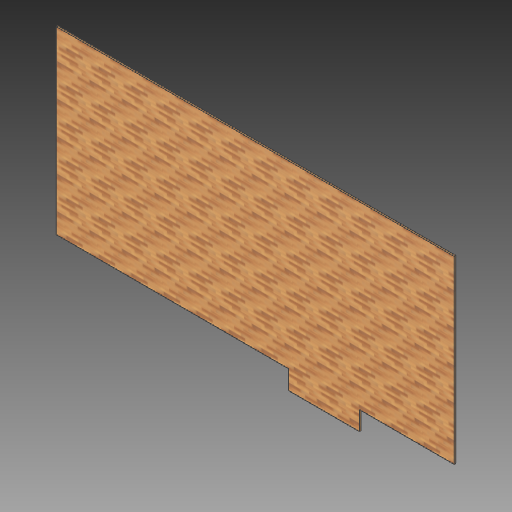
# Autodesk Inventor part: Пол гостиной
Saved by Autodesk Inventor 2019 (Build 230136000, 136)
## iProperties
Created: 2018-09-19
Part Number: Пол гостиной
Material: Деревянные полы
Document SubType Name: Modeling
Designer: Андреев Н.Л.
Density: 0.673 g/cm^3
Appearance: Бук — гальяно
Author: Андреев Н.Л.
Autodesk Inventor part; units mm, degrees
ref_plane "YZ Plane" through (0, 0, 0) normal (1, 0, 0) x (0, 1, 0)
ref_plane "XZ Plane" through (0, 0, 0) normal (0, 1, 0) x (-1, 0, 0)
ref_plane "XY Plane" through (0, 0, 0) normal (0, 0, 1) x (1, 0, 0)
sketch "Эскиз1" plane through (0, 0, 0) normal (0, 0, 1) x (1, 0, 0)
  line L0 (23007.3162, 20272.69) -> (23007.3162, 20672.69) construction
  line L1 (25007.3162, 20672.69) -> (23007.3162, 20672.69) construction
  line L2 (25007.3162, 20272.69) -> (25007.3162, 20672.69) construction
  line L3 (23007.3162, 20272.69) -> (25007.3162, 20272.69) construction
  line L4 (21507.3162, 20672.69) -> (21507.3162, 20272.69) construction
  line L5 (19507.3162, 20272.69) -> (21507.3162, 20272.69) construction
  line L6 (19507.3162, 20672.69) -> (19507.3162, 20272.69) construction
  line L7 (21507.3162, 20672.69) -> (19507.3162, 20672.69) construction
  line L8 (28307.3162, 15072.69) -> (28307.3162, 14672.69) construction
  line L9 (27607.3162, 14672.69) -> (28307.3162, 14672.69) construction
  line L10 (27607.3162, 15072.69) -> (27607.3162, 14672.69) construction
  line L11 (26657.3162, 15072.69) -> (27607.3162, 15072.69) construction
  line L12 (26657.3162, 15072.69) -> (26657.3162, 15472.69) construction
  line L13 (27607.3162, 15472.69) -> (26657.3162, 15472.69) construction
  line L14 (27607.3162, 23072.69) -> (27607.3162, 15472.69) construction
  line L15 (25407.3162, 23072.69) -> (27607.3162, 23072.69) construction
  line L16 (25407.3162, 20072.69) -> (25407.3162, 23072.69) construction
  line L17 (25407.3162, 20072.69) -> (25007.3162, 20072.69) construction
  line L18 (25007.3162, 14072.69) -> (25007.3162, 17872.69) construction
  line L19 (25007.3162, 24472.69) -> (16607.3162, 24472.69) construction
  line L20 (16607.3162, 24472.69) -> (16607.3162, 20672.69) construction
  line L21 (19507.3162, 20672.69) -> (16607.3162, 20672.69) construction
  line L22 (19507.3162, 20272.69) -> (19507.3162, 20672.69) construction
  line L23 (16607.3162, 20272.69) -> (19507.3162, 20272.69) construction
  line L24 (16607.3162, 20272.69) -> (16607.3162, 18272.69) construction
  line L25 (19607.3162, 18272.69) -> (16607.3162, 18272.69) construction
  line L26 (19607.3162, 18272.69) -> (19607.3162, 17872.69) construction
  line L27 (16607.3162, 17872.69) -> (19607.3162, 17872.69) construction
  line L28 (16607.3162, 17872.69) -> (16607.3162, 14072.69) construction
  line L29 (16607.3162, 14072.69) -> (25007.3162, 14072.69) construction
  line L30 (23857.3162, 17872.69) -> (25007.3162, 17872.69) construction
  line L31 (23857.3162, 17872.69) -> (23857.3162, 18272.69) construction
  line L32 (25007.3162, 18272.69) -> (23857.3162, 18272.69) construction
  line L33 (25007.3162, 18272.69) -> (25007.3162, 18572.69) construction
  line L34 (25007.3162, 18572.69) -> (25407.3162, 18572.69) construction
  line L35 (25407.3162, 15472.69) -> (25407.3162, 18572.69) construction
  line L36 (25657.3162, 15472.69) -> (25407.3162, 15472.69) construction
  line L37 (25657.3162, 15472.69) -> (25657.3162, 15072.69) construction
  line L38 (25407.3162, 15072.69) -> (25657.3162, 15072.69) construction
  line L39 (25407.3162, 13672.69) -> (25407.3162, 15072.69) construction
  line L40 (16207.3162, 13672.69) -> (25407.3162, 13672.69) construction
  line L41 (16207.3162, 15072.69) -> (16207.3162, 13672.69) construction
  line L42 (15957.3162, 15072.69) -> (16207.3162, 15072.69) construction
  line L43 (15957.3162, 15072.69) -> (15957.3162, 15472.69) construction
  line L44 (16207.3162, 15472.69) -> (15957.3162, 15472.69) construction
  line L45 (16207.3162, 23472.69) -> (16207.3162, 15472.69) construction
  line L46 (14007.3162, 23472.69) -> (16207.3162, 23472.69) construction
  line L47 (14007.3162, 20472.69) -> (14007.3162, 23472.69) construction
  line L48 (14007.3162, 20472.69) -> (13607.3162, 20472.69) construction
  line L49 (13607.3162, 20472.69) -> (13607.3162, 23472.69) construction
  line L50 (13607.3162, 23472.69) -> (8007.3162, 23472.69) construction
  line L51 (8007.3162, 23472.69) -> (8007.3162, 15072.69) construction
  line L52 (8007.3162, 15072.69) -> (13607.3162, 15072.69) construction
  line L53 (13607.3162, 15072.69) -> (13607.3162, 18072.69) construction
  line L54 (13607.3162, 18072.69) -> (14007.3162, 18072.69) construction
  line L55 (14007.3162, 15472.69) -> (14007.3162, 18072.69) construction
  line L56 (14957.3162, 15472.69) -> (14007.3162, 15472.69) construction
  line L57 (14957.3162, 15472.69) -> (14957.3162, 15072.69) construction
  line L58 (14007.3162, 15072.69) -> (14957.3162, 15072.69) construction
  line L59 (14007.3162, 14672.69) -> (14007.3162, 15072.69) construction
  line L60 (7607.3162, 14672.69) -> (14007.3162, 14672.69) construction
  line L61 (7607.3162, 23872.69) -> (7607.3162, 14672.69) construction
  line L62 (16207.3162, 23872.69) -> (7607.3162, 23872.69) construction
  line L63 (16207.3162, 24872.69) -> (16207.3162, 23872.69) construction
  line L64 (25407.3162, 24872.69) -> (16207.3162, 24872.69) construction
  line L65 (25407.3162, 23472.69) -> (25407.3162, 24872.69) construction
  line L66 (27607.3162, 23472.69) -> (25407.3162, 23472.69) construction
  line L67 (27607.3162, 23872.69) -> (27607.3162, 23472.69) construction
  line L68 (29607.3162, 23872.69) -> (27607.3162, 23872.69) construction
  line L69 (29607.3162, 23872.69) -> (29607.3162, 23472.69) construction
  line L70 (29607.3162, 23472.69) -> (28007.3162, 23472.69) construction
  line L71 (28007.3162, 23472.69) -> (28007.3162, 15072.69) construction
  line L72 (28007.3162, 15072.69) -> (28307.3162, 15072.69) construction
  line L73 (25007.3162, 20672.69) -> (25007.3162, 24472.69)
  line L74 (16607.3162, 24472.69) -> (25007.3162, 24472.69)
  line L75 (16607.3162, 24472.69) -> (16607.3162, 20672.69)
  line L76 (16607.3162, 20672.69) -> (21507.3162, 20672.69)
  line L77 (21507.3162, 20672.69) -> (21507.3162, 20272.69)
  line L78 (21507.3162, 20272.69) -> (23007.3162, 20272.69)
  line L79 (23007.3162, 20272.69) -> (23007.3162, 20672.69)
  line L80 (23007.3162, 20672.69) -> (25007.3162, 20672.69)
  line L81 (25307.3162, 23070.3586) -> (25007.3162, 23070.3586) projected
  line L82 (25007.3162, 23070.3586) -> (25007.3162, 24472.69) projected
  line L83 (25007.3162, 20072.69) -> (25007.3162, 22270.3586) projected
  line L84 (25007.3162, 22270.3586) -> (25307.3162, 22270.3586) projected
  line L85 (25307.3162, 22270.3586) -> (25307.3162, 23070.3586) projected
  point P0 (0, 0)
  constraints: 16 end point, 5 perpendicular, 3 collinear
extrude "Выдавливание1" add sketch "Эскиз1" along normal blind 32 contours L80 L79 L78 L77 L76 L75 L74 L73
